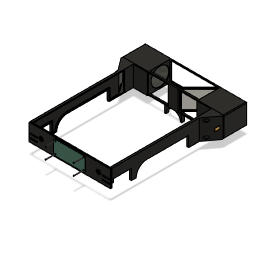
ARGlass (Autodesk Fusion 360 design; units mm, degrees)
Autodesk Fusion 360 part; units mm, degrees
note: some values were not read from the file. Chosen so that the rebuilt part matches the saved one: a direction; which face or edge a step refers to. Set by a fixed rule: which sketch regions a step uses; the direction of a hole.
(part 1 of 2)
sketch "スケッチ1" plane through (0, 0, 0) normal (0, 1, 0) x (1, 0, 0) in component "Display"
  line L0 (0, 0) -> (26.85, 0)
  line L1 (26.85, 0) -> (26.85, -29.55)
  line L2 (26.85, -29.55) -> (0, -29.55)
  line L3 (0, -29.55) -> (0, 0)
  dimension "d1" = 26.85
  dimension "d2" = 29.55
  constraint horizontal L0
  constraint vertical L1
  constraint horizontal L2
  constraint vertical L3
  constraint coincident L0.start L3.end
  measures "d1" distance of L0.start L0.end
  measures "d2" distance of L0.start L2.end
extrude "押し出し1" add sketch "スケッチ1" along normal blind 1.37 makes body 1 in component "Display"
sketch "スケッチ2" plane through (0, 1.37, 0) normal (0, 1, 0) x (-1, 0, 0) in component "Display"
  line L0 (0, 29.55) -> (-26.85, 29.55)
  line L1 (-26.85, 29.55) -> (-26.85, 0)
  line L2 (-26.85, 0) -> (0, 0)
  line L3 (0, 0) -> (0, 29.55)
  line L4 (-0.52, 0.55) -> (-26.32, 0.55)
  line L5 (-26.32, 0.55) -> (-26.32, 28.95)
  line L6 (-26.32, 28.95) -> (-0.52, 28.95)
  line L7 (-0.52, 28.95) -> (-0.52, 0.55)
  dimension "d5" = 25.8
  dimension "d6" = 28.4
  dimension "d7" = 0.55
  dimension "d8" = 0.53
  constraint horizontal L4
  constraint vertical L5
  constraint horizontal L6
  constraint vertical L7
  measures "d5" distance of L4.start L4.end
  measures "d6" distance of L4.start L6.end
  measures "d7" distance of L2 L4
  measures "d8" distance of L1 L5
extrude "押し出し2" add sketch "スケッチ2" along normal blind 0.36 separate body contours L4 L5 L6 L7 makes body 2 in component "Display"
sketch "スケッチ3" plane through (0, 1.37, 0) normal (0, 1, 0) x (-1, 0, 0) in component "Display"
  line L0 (0, 29.55) -> (-26.85, 29.55)
  line L1 (-26.85, 29.55) -> (-26.85, 0)
  line L2 (-26.85, 0) -> (0, 0)
  line L3 (0, 0) -> (0, 29.55)
  line L4 (-5.05, 28.95) -> (-23.05, 28.95)
  line L5 (-23.05, 28.95) -> (-23.05, 33.95)
  line L6 (-5.05, 33.95) -> (-5.05, 28.95)
  line L7 (-5.05, 33.95) -> (-10.8, 33.95)
  line L8 (-10.8, 33.95) -> (-10.8, 49.55)
  line L9 (-10.8, 49.55) -> (-17.3, 49.55)
  line L10 (-17.3, 49.55) -> (-17.3, 33.95)
  line L11 (-17.3, 33.95) -> (-23.05, 33.95)
  line L12 (-14.05, 28.95) -> (-14.05, 49.55) construction
  line L13 (-0.52, 28.95) -> (-26.32, 28.95)
  dimension "d11" = 6.5
  dimension "d12" = 10.8
  dimension "d13" = 18
  dimension "d14" = 20
  dimension "d15" = 5
  constraint horizontal L4
  constraint vertical L5
  constraint vertical L6
  constraint perpendicular L6 L7
  constraint perpendicular L7 L8
  constraint perpendicular L6 L9
  constraint perpendicular L9 L10
  constraint perpendicular L5 L11
  constraint midpoint L4 L12.start
  constraint midpoint L9 L12.end
  constraint vertical L12
  constraint collinear L4 L13
  constraint collinear L7 L11
  measures "d11" distance of L8.end L9.end
  measures "d12" distance of L3 L8
  measures "d13" distance of L5 L6
  measures "d14" distance of L0 L9
  measures "d15" distance of L4.end L5.end
extrude "押し出し3" add sketch "スケッチ3" against normal blind 0.3 separate body contours L0 L5 L6 L7 L8 L9 L10 L11 makes body 3 in component "Display"
sketch "スケッチ1 (2)" plane through (0, 0, 0) normal (0, 0, 1) x (1, 0, 0) in component "Lens"
  arc A0 (18.375, 0.3703) -> (0, 1.5) centre (0, -148.5) ccw
  line L0 (0, 0) -> (25.0146, 0) construction
  arc A1 (0, -1.5) -> (18.375, -0.3703) centre (0, 148.5) ccw
  line L1 (18.375, -0.3703) -> (18.375, 0.3703)
  line L2 (0, -1.5) -> (0, 1.5)
  line L3 (0, 1.5) -> (-2.5, 1.5) construction
  dimension "d18" = 150
  dimension "d19" = 3
  dimension "d20" = 18.375
  constraint coincident L0.start origin
  constraint horizontal L0
  constraint symmetric A0.start L0 A1.end
  constraint symmetric A0.end L0 A1.start
  constraint symmetric A0 L0 A1
  constraint coincident L0.start L2
  constraint perpendicular L2 L3
  constraint tangent A0 L3
  measures "d18" radius of A0
  measures "d19" distance of A0.end A1.start
  measures "d20" distance of L0.start L1
revolve "回転1" add sketch "スケッチ1 (2)" angle 360 about axis through (0, 1.75, 0) along (0, 1, 0) separate body makes body 4 in component "Lens"
sketch "スケッチ1 (3)" plane through (0, 0, 0) normal (0, 1, 0) x (1, 0, 0) in component "HalfMirror"
  line L0 (0, 0) -> (38, 0)
  line L1 (38, 0) -> (38, -54)
  line L2 (38, -54) -> (0, -54)
  line L3 (0, -54) -> (0, 0)
  dimension "d80" = 38
  dimension "d81" = 54
  constraint horizontal L0
  constraint vertical L1
  constraint horizontal L2
  constraint vertical L3
  constraint coincident L0.start L3.end
  measures "d80" distance of L0.start L0.end
  measures "d81" distance of L0.start L2.end
extrude "押し出し1'" add sketch "スケッチ1 (3)" along normal blind 0.5 separate body makes body 5 in component "HalfMirror"
sketch "スケッチ1 (4)" plane through (0, 0, 0) normal (0, 1, 0) x (1, 0, 0) in component "Pi Zero W"
  line L0 (3, 0) -> (62, 0)
  line L1 (65, -3) -> (65, -27)
  line L2 (62, -30) -> (3, -30)
  line L3 (0, -27) -> (0, -3)
  arc A0 (3, 0) -> (0, -3) centre (3, -3) ccw
  arc A1 (65, -3) -> (62, 0) centre (62, -3) ccw
  arc A2 (62, -30) -> (65, -27) centre (62, -27) ccw
  arc A3 (0, -27) -> (3, -30) centre (3, -27) ccw
  point P0 (65, 0)
  point P1 (0, -30)
  point P2 (3.5, -3.5)
  point P3 (61.5, -3.5)
  point P4 (3.5, -26.5)
  point P5 (61.5, -26.5)
  dimension "d140" = 65
  dimension "d141" = 30
  dimension "d142" = 3
  dimension "d143" = 3.5
  dimension "d144" = 3.5
  dimension "d147" = 58
  dimension "d148" = -23
  constraint horizontal L0
  constraint vertical L1
  constraint horizontal L2
  constraint vertical L3
  constraint coincident origin L0
  constraint coincident origin L3
  constraint tangent L0 A0
  constraint tangent L3 A0
  constraint coincident P0 L0
  constraint coincident P0 L1
  constraint tangent L0 A1
  constraint tangent L1 A1
  constraint equal A0 A1
  constraint tangent L1 A2
  constraint tangent L2 A2
  constraint equal A0 A2
  constraint coincident P1 L2
  constraint coincident P1 L3
  constraint tangent L2 A3
  constraint tangent L3 A3
  constraint equal A0 A3
  measures "d140" distance of origin P0
  measures "d141" distance of origin P1
  measures "d142" radius of A0
  measures "d143" distance of L0 P2
  measures "d144" distance of L3 P2
extrude "押し出し1''" add sketch "スケッチ1 (4)" along normal blind 1 separate body makes body 6 in component "Pi Zero W"
hole "穴1" at (3.5, 0, 26.5) at (3.5, 0, 3.5) at (61.5, 0, 3.5) at (61.5, 0, 26.5) direction (0, 1, 0) diameter 2.5 end through all bodies 6 in component "Pi Zero W"
sketch "スケッチ1 (5)" plane through (0, 0, 0) normal (0, 1, 0) x (1, 0, 0) in component "FrontUnit"
  line L0 (0, 3) -> (7.1716, 3)
  line L1 (0, 0) -> (0, 3)
  line L2 (49.1716, 45) -> (52.1716, 48)
  line L3 (103, 0) -> (0, 0)
  line L4 (53, 46) -> (53, 3)
  line L5 (10, 3) -> (53, 3)
  line L6 (103, 0) -> (103, 48)
  line L7 (52.1716, 48) -> (103, 48)
  line L8 (10, 3) -> (53, 46)
  line L9 (31.5, 24.5) -> (31.5, 0) construction
  line L10 (53, 46) -> (50.1716, 46) construction
  line L11 (52.1716, 48) -> (0, 48)
  line L12 (0, 48) -> (0, 45)
  line L13 (0, 45) -> (49.1716, 45)
  line L14 (7.1716, 3) -> (49.1716, 45)
  dimension "d23" = 3
  dimension "d24" = 31.5
  dimension "d27" = 43
  dimension "d28" = 2
  dimension "d29" = 50
  dimension "d55" = 3
  dimension "d56" = 45
  dimension "d57" = 2
  constraint horizontal L0
  constraint horizontal L3
  constraint vertical L1
  constraint perpendicular L4 L5
  constraint perpendicular L6 L7
  constraint horizontal L7
  constraint horizontal L5
  constraint coincident L1.start L3.end
  constraint collinear L0 L5
  constraint midpoint L8 L9.start
  constraint coincident L3 L9.end
  constraint perpendicular L3 L9
  constraint coincident L2 L10.end
  constraint horizontal L10
  constraint coincident L4.start L10
  constraint perpendicular L4 L11
  constraint perpendicular L11 L12
  constraint perpendicular L12 L13
  constraint collinear L1 L12
  constraint parallel L8 L14
  constraint parallel L2 L8
  constraint coincident L4.start L8.end
  measures "d23" distance of L0.start L1.start
  measures "d24" distance of L1 L9
  measures "d27" distance of L4.start L4.end
  measures "d28" distance of L4.start L7
  measures "d29" distance of L4 L6
  measures "d55" distance of L11.end L12.end
  measures "d56" angle of L5 L8
  measures "d57" distance of L8 L14
extrude "押し出し1'''" add sketch "スケッチ1 (5)" along normal blind 2 separate body makes body 7 in component "FrontUnit"
sketch "スケッチ2 (2)" plane through (53, 0, 0) normal (-1, 0, 0) x (0, 0, 1) in component "FrontUnit"
  line L0 (-46, 0) -> (-3, 0)
  line L1 (-3, 0) -> (-3, 2)
  line L2 (-3, 2) -> (-46, 2)
  line L3 (-46, 2) -> (-3, 2)
  line L4 (-24.5, 2) -> (-24.5, 21) construction
  line L5 (-48, 40) -> (-48, 2)
  line L6 (-48, 2) -> (-46, 2)
  line L7 (0, 40) -> (0, 2)
  line L8 (-3, 2) -> (0, 2)
  circle A0 centre (-24.5, 21) radius 19
  line L9 (-48, 40) -> (0, 40)
  line L10 (-46, 2) -> (-46, 0)
  point P0 (0, 2)
  point P1 (-48, 2)
  dimension "d36" = 38
  constraint midpoint L3 L4.start
  constraint vertical L4
  constraint coincident L2.end L3.start
  constraint perpendicular L3 L7
  constraint coincident L1.end L2.start
  constraint perpendicular L7 L8
  constraint coincident P0 L7.end
  constraint coincident L4.end A0.centre
  constraint tangent L2 A0
  constraint tangent A0 L9
  constraint horizontal L9
  constraint vertical L5
  constraint coincident L5 P1
  constraint coincident L6 P1
  measures "d36" diameter of A0
extrude "押し出し2'" add sketch "スケッチ2 (2)" along normal blind 2 contours L2 L3 L5 L6 A0 L9 | L2 L3 L7 L8 A0 L9 bodies 7 in component "FrontUnit"
sketch "スケッチ3 (2)" plane through (103, 0, 0) normal (1, 0, 0) x (0, 0, -1) in component "FrontUnit"
  line L0 (0, 0) -> (48, 0)
  line L1 (48, 0) -> (48, 2)
  line L2 (48, 2) -> (0, 2)
  line L3 (0, 2) -> (0, 0)
  line L4 (0, 0) -> (48, 0)
  line L5 (48, 0) -> (48, 40)
  line L6 (48, 40) -> (0, 40)
  line L7 (0, 40) -> (0, 0)
  point P0 (48, 40)
  constraint horizontal L4
  constraint vertical L5
  constraint horizontal L6
  constraint vertical L7
  constraint coincident L0.start L3.end
  constraint coincident P0 L5.end
extrude "押し出し3'" add sketch "スケッチ3 (2)" along normal blind 2 bodies 7 in component "FrontUnit"
sketch "スケッチ4" plane through (103, 0, 0) normal (-1, 0, 0) x (0, 0, 1) in component "FrontUnit"
  line L0 (-48, 2) -> (0, 2)
  line L1 (0, 2) -> (0, 40)
  line L2 (0, 40) -> (-48, 40)
  line L3 (-48, 40) -> (-48, 2)
  line L4 (-15.205, 34.675) -> (-45.255, 34.675)
  line L5 (-45.255, 34.675) -> (-45.255, 7.325)
  line L6 (-45.255, 7.325) -> (-15.205, 7.325)
  line L7 (-15.205, 7.325) -> (-15.205, 34.675) construction
  line L8 (-15.205, 34.675) -> (-45.255, 7.325) construction
  line L9 (-45.255, 34.675) -> (-15.205, 7.325) construction
  arc A0 (-24.5, 2) -> (-24.5, 40) centre (-24.5, 21) ccw construction
  arc A1 (-24.5, 40) -> (-24.5, 2) centre (-24.5, 21) ccw construction
  line L10 (-15.205, 34.675) -> (0, 34.675)
  line L11 (-15.205, 7.325) -> (0, 7.325)
  line L12 (-30.23, 21) -> (-24.5, 21) construction
  point P0 (-30.23, 21)
  dimension "d39" = 30.05
  dimension "d40" = 27.35
  dimension "d88" = 5.73
  constraint horizontal L4
  constraint perpendicular L4 L5
  constraint parallel L4 L6
  constraint parallel L5 L7
  constraint coincident L8 P0
  constraint coincident L9 P0
  constraint coincident L1 L10.end
  constraint perpendicular L1 L10
  constraint coincident L1 L11.end
  constraint perpendicular L1 L11
  constraint coincident P0 L12.start
  constraint coincident A0.centre A1.centre
  constraint horizontal L12
  measures "d39" distance of L5.end L6.end
  measures "d40" distance of L4.end L5.end
  measures "d88" distance of P0 A0.centre
extrude "押し出し4" add sketch "スケッチ4" along normal blind 1.3 contours L0 L1 L2 L3 L4 L5 L6 L10 L11 bodies 7 in component "FrontUnit"
sketch "スケッチ5" plane through (0, 0, -48) normal (0, 0, -1) x (-1, 0, 0) in component "FrontUnit"
  line L0 (-105, 0) -> (0, 0)
  line L1 (0, 2) -> (-51, 2)
  line L2 (-51, 2) -> (-51, 40)
  line L3 (-51, 40) -> (-53, 40)
  line L4 (-53, 40) -> (-53, 2)
  line L5 (-53, 2) -> (-101.7, 2)
  line L6 (-101.7, 2) -> (-101.7, 40)
  line L7 (-101.7, 40) -> (-105, 40)
  line L8 (-105, 40) -> (-105, 0)
  line L9 (-101.7, 40) -> (-101.7, 2)
  line L10 (-101.7, 2) -> (-53, 2)
  line L11 (-53, 40) -> (-53, 2)
  line L12 (-101.7, 40) -> (-53, 40)
  line L13 (0, 0) -> (0, 2)
  constraint coincident L6.end L7.start
  constraint coincident L3.end L4.start
extrude "押し出し5" add sketch "スケッチ5" against normal blind 2 contours L4 L5 L6 L9 L10 L11 L12 bodies 7 in component "FrontUnit"
sketch "スケッチ6" plane through (0, 40, 0) normal (0, 1, 0) x (-1, 0, 0) in component "FrontUnit"
  line L0 (-105, -48) -> (-51, -48)
  line L1 (-51, -48) -> (-51, -24.5)
  line L2 (-51, -24.5) -> (-53, -24.5)
  line L3 (-53, -24.5) -> (-53, -46)
  line L4 (-53, -46) -> (-101.7, -46)
  line L5 (-101.7, -46) -> (-101.7, 0)
  line L6 (-101.7, 0) -> (-105, 0)
  line L7 (-105, 0) -> (-105, -48)
  line L8 (-105, -48) -> (-51, -48)
  line L9 (-105, -48) -> (-105, 0)
  line L10 (-51, -24.5) -> (-51, -48)
  line L11 (-51, 0) -> (-51, -24.5)
  line L12 (-53, 0) -> (-51, 0)
  line L13 (-53, 0) -> (-101.7, 0)
  line L14 (-105, 0) -> (-101.7, 0)
extrude "押し出し6" add sketch "スケッチ6" along normal blind 2 bodies 7 in component "FrontUnit"
sketch "スケッチ7" plane through (0, 2, 0) normal (0, -1, 0) x (1, 0, 0) in component "FrontUnit"
  line L0 (53, -3) -> (51, -3)
  line L1 (51, -3) -> (51, -24.5)
  line L2 (53, -24.5) -> (53, -3)
  line L3 (51, -24.5) -> (51, -3)
  line L4 (53, -46) -> (53, -3)
  line L5 (51, -44) -> (51, -24.5)
  line L6 (53, -46) -> (51, -44)
  line L7 (51, -3) -> (53, -3)
  constraint coincident L4.start L6.start
  constraint coincident L5.start L6.end
  constraint coincident L0.end L1.start
  constraint coincident L0.start L2.end
extrude "押し出し7" add sketch "スケッチ7" along normal blind 2 bodies 7 in component "FrontUnit"
sketch "スケッチ8" plane through (0, 42, 0) normal (0, 1, 0) x (-1, 0, 0) in component "FrontUnit"
  line L0 (-105, -48) -> (-51, -48)
  line L1 (-51, -48) -> (-51, 0)
  line L2 (-51, 0) -> (-105, 0)
  line L3 (-105, 0) -> (-105, -48)
  line L4 (-51, -44) -> (-51, -48)
  line L5 (-51, -48) -> (0, -48)
  line L6 (-7.1716, -3) -> (0, -3)
  line L7 (0, -3) -> (0, 0)
  line L8 (0, 0) -> (-51, 0)
  line L9 (-51, 0) -> (-51, -3)
  line L10 (-51, -3) -> (-10, -3)
  line L11 (0, -48) -> (0, -45)
  line L12 (0, -45) -> (-49.1716, -45)
  line L13 (-49.1716, -45) -> (-7.1716, -3)
  line L14 (-10, -3) -> (-51, -44)
extrude "押し出し8" add sketch "スケッチ8" against normal blind 2 contours L1 L4 L5 L6 L7 L8 L9 L10 L11 L12 L13 L14 bodies 7 in component "FrontUnit"
sketch "スケッチ9" plane through (0, 2, 0) normal (0, 1, 0) x (-1, 0, 0) in component "FrontUnit"
  line L0 (-51, -44) -> (-51, -48)
  line L1 (-51, -48) -> (0, -48)
  line L2 (-7.1716, -3) -> (0, -3)
  line L3 (0, -3) -> (0, 0)
  line L4 (0, 0) -> (-51, 0)
  line L5 (-51, 0) -> (-51, -3)
  line L6 (-51, -3) -> (-10, -3)
  line L7 (0, 0) -> (-10, 0)
  line L8 (-10, 0) -> (-10, -3)
  line L9 (-10, -3) -> (0, -3)
  line L10 (0, -3) -> (0, 0)
  line L11 (0, -48) -> (0, -45)
  line L12 (0, -45) -> (-49.1716, -45)
  line L13 (-49.1716, -45) -> (-7.1716, -3)
  line L14 (-10, -3) -> (-51, -44)
  dimension "d51" = 10
  dimension "d52" = 3
  constraint horizontal L7
  constraint vertical L8
  constraint horizontal L9
  constraint vertical L10
  constraint coincident L3.end L4.start
  measures "d51" distance of L6.end L2.end
  measures "d52" distance of L3.end L2.end
extrude "押し出し9" add sketch "スケッチ9" along normal up to near side of body 7 contours L2 L3 L4 L7 L8 L9 L10 bodies 7 in component "FrontUnit"
sketch "スケッチ10" plane through (3.5, 0, 3.5) normal (0.707107, 0, 0.707107) x (0.707107, 0, -0.707107) in component "FrontUnit"
  line L0 (67.1751, 42) -> (9.1924, 42)
  line L1 (9.1924, 42) -> (9.1924, 40)
  line L2 (9.1924, 40) -> (67.1751, 40)
  line L3 (67.1751, 40) -> (67.1751, 42)
  line L4 (12.1924, 39) -> (64.1751, 39)
  line L5 (64.1751, 39) -> (64.1751, 3)
  line L6 (64.1751, 3) -> (12.1924, 3)
  line L7 (12.1924, 3) -> (12.1924, 39)
  line L8 (9.1924, 42) -> (67.1751, 42)
  line L9 (9.1924, 0) -> (67.1751, 0)
  line L10 (6.1924, 42) -> (6.1924, 0)
  line L11 (6.1924, 0) -> (9.1924, 0)
  line L12 (6.1924, 42) -> (9.1924, 42)
  line L13 (67.1751, 42) -> (70.1751, 42)
  line L14 (70.1751, 42) -> (70.1751, 0)
  line L15 (70.1751, 0) -> (67.1751, 0)
  dimension "d62" = 3
  dimension "d63" = 3
  dimension "d64" = 3
  dimension "d65" = 3
  dimension "d68" = 3
  dimension "d69" = 3
  constraint horizontal L4
  constraint vertical L5
  constraint horizontal L6
  constraint vertical L7
  constraint vertical L10
  constraint coincident L9.start L11.end
  constraint perpendicular L10 L11
  constraint coincident L0.end L1.start
  constraint horizontal L12
  constraint coincident L0.start L3.end
  constraint perpendicular L3 L13
  constraint perpendicular L8 L14
  constraint coincident L9.end L15.end
  constraint perpendicular L14 L15
  measures "d62" distance of L0 L4
  measures "d63" distance of L6 L9
  measures "d64" distance of L10.start L0.end
  measures "d65" distance of L0.start L13.end
  measures "d68" distance of L7 L0.end
  measures "d69" distance of L5 L0.start
extrude "押し出し10" add sketch "スケッチ10" against normal blind 2 bodies 7 in component "FrontUnit"
sketch "スケッチ12" plane through (3.5, 0, 3.5) normal (0.707107, 0, 0.707107) x (0.707107, 0, -0.707107) in component "FrontUnit"
  line L0 (64.1751, 3) -> (12.1924, 3)
  line L1 (12.1924, 3) -> (12.1924, 39)
  line L2 (12.1924, 39) -> (64.1751, 39)
  line L3 (64.1751, 39) -> (64.1751, 3)
  line L4 (67.1751, 0) -> (67.1751, 42)
  line L5 (67.1751, 42) -> (9.1924, 42)
  line L6 (9.1924, 42) -> (9.1924, 40)
  line L7 (9.1924, 40) -> (9.1924, 2)
  line L8 (9.1924, 2) -> (9.1924, 0)
  line L9 (9.1924, 0) -> (67.1751, 0)
  line L10 (10.6924, 40.5) -> (65.6751, 40.5)
  line L11 (65.6751, 40.5) -> (65.6751, 1.5)
  line L12 (65.6751, 1.5) -> (10.6924, 1.5)
  line L13 (10.6924, 1.5) -> (10.6924, 40.5)
  line L14 (12.1924, 39) -> (12.1924, 3)
  line L15 (12.1924, 39) -> (64.1751, 39)
  line L16 (64.1751, 3) -> (64.1751, 39)
  line L17 (64.1751, 3) -> (12.1924, 3)
  line L18 (64.1751, 3) -> (64.1751, 39)
  line L19 (64.1751, 39) -> (64.1751, 3)
  dimension "d235" = 1.5
  dimension "d236" = 1.5
  dimension "d237" = 1.5
  dimension "d238" = 1.5
  constraint horizontal L10
  constraint vertical L11
  constraint horizontal L12
  constraint vertical L13
  measures "d235" distance of L10 L15
  measures "d236" distance of L13 L14
  measures "d237" distance of L11 L19
  measures "d238" distance of L0 L12
extrude "押し出し13" cut sketch "スケッチ12" against normal blind 0.5 contours L10 L11 L12 L13 bodies 7 in component "FrontUnit"
sketch "スケッチ11" plane through (0, 0, 0) normal (0, 0, 1) x (1, 0, 0) in component "FrontUnit"
  line L0 (10, 40) -> (51, 40)
  line L1 (51, 40) -> (51, 2)
  line L2 (51, 2) -> (10, 2)
  line L3 (10, 2) -> (10, 40)
  line L4 (0, 42) -> (0, 0)
  line L5 (0, 0) -> (105, 0)
  line L6 (105, 0) -> (105, 42)
  line L7 (105, 42) -> (0, 42)
  line L8 (53, 40) -> (101.7, 40)
  line L9 (101.7, 40) -> (101.7, 34.675)
  line L10 (101.7, 34.675) -> (103, 34.675)
  line L11 (103, 34.675) -> (103, 7.325)
  line L12 (103, 7.325) -> (101.7, 7.325)
  line L13 (101.7, 7.325) -> (101.7, 2)
  line L14 (101.7, 2) -> (53, 2)
  line L15 (53, 2) -> (53, 40)
  line L16 (85.3, 40) -> (94.7, 40)
  line L17 (94.7, 40) -> (94.7, 36.15)
  line L18 (85.3, 36.15) -> (85.3, 40)
  arc A0 (85.3, 36.15) -> (94.7, 36.15) centre (90, 36.15) ccw
  line L19 (91.6454, 33.3) -> (93.2909, 36.15)
  line L20 (93.2909, 36.15) -> (91.6454, 39)
  line L21 (91.6454, 39) -> (88.3546, 39)
  line L22 (88.3546, 39) -> (86.7091, 36.15)
  line L23 (86.7091, 36.15) -> (88.3546, 33.3)
  line L24 (88.3546, 33.3) -> (91.6454, 33.3)
  line L25 (0, 21) -> (105, 21) construction
  line L26 (85.3, 5.85) -> (85.3, 2)
  arc A1 (94.7, 5.85) -> (85.3, 5.85) centre (90, 5.85) ccw
  line L27 (94.7, 2) -> (94.7, 5.85)
  line L28 (85.3, 2) -> (94.7, 2)
  line L29 (93.2909, 5.85) -> (91.6454, 3)
  line L30 (91.6454, 8.7) -> (93.2909, 5.85)
  line L31 (88.3546, 8.7) -> (91.6454, 8.7)
  line L32 (86.7091, 5.85) -> (88.3546, 8.7)
  line L33 (88.3546, 3) -> (86.7091, 5.85)
  line L34 (91.6454, 3) -> (88.3546, 3)
  point P0 (90, 36.15)
  dimension "d89" = 5.7
  dimension "d90" = 1
  dimension "d91" = 90
  dimension "d92" = 9.4
  constraint horizontal L16
  constraint vertical L17
  constraint vertical L18
  constraint coincident L8 L16.start
  constraint tangent L18 A0
  constraint tangent L17 A0
  constraint coincident P0 A0.centre
  constraint midpoint L4 L25.start
  constraint midpoint L6 L25.end
  constraint symmetric L16.start L25 L26.end
  constraint symmetric L16.end L25 L27.start
  constraint symmetric L17.end L25 A1.start
  constraint symmetric L18.start L25 L26.start
  constraint symmetric A0 L25 A1
  constraint symmetric L19.start L25 L30.start
  constraint symmetric L19.end L25 L29.start
  constraint symmetric L20.end L25 L29.end
  constraint symmetric L21.end L25 L33.start
  constraint symmetric L22.end L25 L32.start
  constraint symmetric L23.end L25 L31.start
  measures "d89" distance of L21 L24
  measures "d90" distance of L16 L21
  measures "d91" distance of L4 P0
  measures "d92" distance of L16.start L16.end
extrude "押し出し11" add sketch "スケッチ11" against normal blind 4.5 contours L8 L16 L17 L18 A0 | L14 L26 A1 L27 L28 | L19 L20 L21 L22 L23 L24 | L29 L30 L31 L32 L33 L34 bodies 7 in component "FrontUnit"
extrude "押し出し12" cut sketch "スケッチ11" against normal blind 3 contours L19 L20 L21 L22 L23 L24 | L29 L30 L31 L32 L33 L34 bodies 7 in component "FrontUnit"
ref_plane "作業平面1" through (80, 0, 0) normal (1, 0, 0) x (0, 1, 0) in component "SideUnit"
sketch "スケッチ1 (6)" plane through (80, 0, 0) normal (1, 0, 0) x (0, 0, -1) in component "SideUnit"
  line L0 (0, 0) -> (-30, 0)
  line L1 (-30, 42) -> (0, 42)
  line L2 (0, 42) -> (0, 0)
  line L3 (0, 42) -> (48, 42) construction
  line L4 (-30, 0) -> (-30, 42)
  dimension "d98" = 30
  constraint horizontal L0
  constraint horizontal L1
  constraint vertical L2
  constraint coincident L0.start L2.end
  constraint coincident L1.end L2.start
  constraint vertical L4
  measures "d98" distance of L0.start L0.end
extrude "押し出し1''''" add sketch "スケッチ1 (6)" along normal blind 2 separate body makes body 8 in component "SideUnit"
sketch "スケッチ2 (3)" plane through (0, 0, 0) normal (0, 0, 1) x (1, 0, 0) in component "SideUnit"
  line L0 (93.2909, 36.15) -> (91.6454, 33.3)
  line L1 (91.6454, 33.3) -> (88.3546, 33.3)
  line L2 (88.3546, 33.3) -> (86.7091, 36.15)
  line L3 (86.7091, 36.15) -> (88.3546, 39)
  line L4 (88.3546, 39) -> (91.6454, 39)
  line L5 (91.6454, 39) -> (93.2909, 36.15)
  line L6 (91.6454, 8.7) -> (93.2909, 5.85)
  line L7 (93.2909, 5.85) -> (91.6454, 3)
  line L8 (91.6454, 3) -> (88.3546, 3)
  line L9 (88.3546, 3) -> (86.7091, 5.85)
  line L10 (86.7091, 5.85) -> (88.3546, 8.7)
  line L11 (88.3546, 8.7) -> (91.6454, 8.7)
  line L12 (10, 40) -> (51, 40)
  line L13 (51, 40) -> (51, 2)
  line L14 (51, 2) -> (10, 2)
  line L15 (10, 2) -> (10, 40)
  line L16 (0, 42) -> (0, 0)
  line L17 (0, 0) -> (105, 0)
  line L18 (105, 0) -> (105, 42)
  line L19 (105, 42) -> (0, 42)
  line L20 (94.7, 40) -> (101.7, 40)
  line L21 (101.7, 40) -> (101.7, 34.675)
  line L22 (101.7, 7.325) -> (101.7, 2)
  line L23 (101.7, 2) -> (94.7, 2)
  line L24 (94.7, 2) -> (94.7, 5.85)
  arc A0 (94.7, 5.85) -> (85.3, 5.85) centre (90, 5.85) ccw
  line L25 (85.3, 5.85) -> (85.3, 2)
  line L26 (85.3, 2) -> (53, 2)
  line L27 (53, 2) -> (53, 40)
  line L28 (53, 40) -> (85.3, 40)
  line L29 (85.3, 40) -> (85.3, 36.15)
  arc A1 (85.3, 36.15) -> (94.7, 36.15) centre (90, 36.15) ccw
  line L30 (94.7, 36.15) -> (94.7, 40)
  line L31 (51, 42) -> (105, 42)
  line L32 (105, 0) -> (51, 0)
  line L33 (51, 0) -> (51, 42)
  line L34 (53, 40) -> (53, 2) construction
  line L35 (105, 0) -> (105, 42)
  line L36 (101.7, 34.675) -> (101.7, 40)
  line L37 (101.7, 2) -> (101.7, 7.325)
  line L38 (53, 40) -> (82, 40)
  line L39 (82, 42) -> (82, 0) construction
  line L40 (53, 2) -> (82, 2)
  line L41 (82, 40) -> (101.7, 40)
  line L42 (82, 2) -> (101.7, 2)
  line L43 (82, 2) -> (82, 40)
  line L44 (101.7, 34.675) -> (101.7, 7.325)
  dimension "d105" = 2
  constraint horizontal L31
  constraint horizontal L32
  constraint vertical L33
  constraint coincident L19 L31.start
  constraint coincident L18.end L19.start
  constraint coincident L17.end L18.start
  constraint coincident L27.end L28.start
  constraint coincident L28 L38.end
  constraint coincident L38.end L39
  constraint coincident L26.end L27.start
  constraint coincident L39 L40.end
  constraint coincident L26 L40.end
  constraint coincident L20.end L21.start
  constraint coincident L22.end L23.start
  constraint coincident L21.end L36.start
  constraint coincident L22.start L37.end
  measures "d105" distance of L33 L34
extrude "押し出し2''" add sketch "スケッチ2 (3)" along normal blind 2 contours L13 L17 L18 L19 L31 L32 L33 L35 | L26 L27 L28 L38 L40 L43 bodies 8 in component "SideUnit"
sketch "スケッチ3 (3)" plane through (0, 0, 0) normal (0, -1, 0) x (1, 0, 0) in component "SideUnit"
  line L0 (82, 2) -> (82, 30)
  line L1 (82, 30) -> (80, 30)
  line L2 (80, 30) -> (80, 2)
  line L3 (80, 2) -> (51, 2)
  line L4 (51, 2) -> (51, 0)
  line L5 (82, 30) -> (82, 2)
  line L6 (105, 2) -> (84, 30)
  line L7 (84, 30) -> (82, 30)
  line L8 (105, 2) -> (82, 2)
  dimension "d108" = 2
  constraint coincident L0.end L1.start
  constraint horizontal L7
  constraint coincident L6.start L8.start
  measures "d108" distance of L6.end L0.end
extrude "押し出し3''" add sketch "スケッチ3 (3)" against normal blind 2 bodies 8 in component "SideUnit"
sketch "スケッチ7 (2)" plane through (0, 42, 0) normal (0, 1, 0) x (-1, 0, 0) in component "SideUnit"
  line L0 (-80, 2) -> (-80, 30)
  line L1 (-80, 30) -> (-82, 30)
  line L2 (-82, 30) -> (-82, 2)
  line L3 (-82, 2) -> (-105, 2)
  line L4 (-105, 2) -> (-105, 0)
  line L5 (-105, 0) -> (-51, 0)
  line L6 (-51, 0) -> (-51, 2)
  line L7 (-51, 2) -> (-80, 2)
  line L8 (-105, 2) -> (-101.7, 2)
  line L9 (-82, 0) -> (-82, 30)
  line L10 (-82, 30) -> (-84, 30)
  line L11 (-84, 30) -> (-105, 2)
  line L12 (-101.7, 0) -> (-82, 0)
  line L13 (-101.7, 2) -> (-101.7, 0)
extrude "押し出し7'" add sketch "スケッチ7 (2)" against normal blind 2 contours L2 L3 L8 L9 L10 L11 bodies 8 in component "SideUnit"
ref_plane "作業平面2" through (82, 0, 0) normal (1, 0, 0) x (0, 1, 0) in component "SideUnit"
sketch "スケッチ10 (2)" plane through (82, 0, 0) normal (1, 0, 0) x (0, 0, -1) in component "SideUnit"
  line L0 (-30, 40) -> (-30, 2)
  line L1 (-30, 42) -> (-30, 40)
  line L2 (-30, 0) -> (-30, 2)
  line L3 (-30, 42) -> (-50, 42)
  line L4 (-50, 42) -> (-50, 0)
  line L5 (-50, 0) -> (-30, 0)
  line L6 (-30, 40) -> (-50, 40)
  line L7 (-30, 2) -> (-50, 2)
  line L8 (-50, 42) -> (-170, 42)
  line L9 (-170, 42) -> (-170, 22)
  line L10 (-138, 24) -> (-50, 24)
  line L11 (-50, 40) -> (-170, 40)
  line L12 (-52, 22) -> (-52, 0)
  line L13 (-52, 0) -> (-50, 0)
  arc A0 (-138, 22) -> (-160, 0) centre (-138, 0) ccw
  line L14 (-160, 22) -> (-160, 0) construction
  line L15 (-160, 0) -> (-52, 0) construction
  line L16 (-160, 0) -> (-170, 0)
  line L17 (-170, 0) -> (-170, 22)
  arc A1 (-138, 24) -> (-161.9165, 2) centre (-138, 0) ccw
  line L18 (-161.9165, 2) -> (-168, 2)
  line L19 (-168, 2) -> (-168, 22)
  line L20 (-170, 22) -> (-168, 22) construction
  line L21 (-138, 22) -> (-50, 22)
  line L22 (-170, 42) -> (-210, 42)
  line L23 (-210, 42) -> (-210, 22)
  line L24 (-210, 22) -> (-170, 22)
  line L25 (-170, 40) -> (-210, 40)
  line L26 (-210, 24) -> (-168, 24)
  line L27 (-168, 22) -> (-168, 24)
  dimension "d126" = 20
  dimension "d132" = 20
  dimension "d133" = 120
  dimension "d134" = 2
  dimension "d137" = 160
  dimension "d138" = 2
  dimension "d139" = 2
  dimension "d168" = 40
  dimension "d169" = 2
  constraint coincident L1.start L3.start
  constraint perpendicular L1 L3
  constraint perpendicular L3 L4
  constraint coincident L2.start L5.end
  constraint perpendicular L2 L5
  constraint coincident L0.start L1.end
  constraint coincident L4 L6.end
  constraint perpendicular L4 L6
  constraint coincident L0.end L2.end
  constraint coincident L4 L7.end
  constraint perpendicular L4 L7
  constraint perpendicular L4 L8
  constraint perpendicular L3 L9
  constraint coincident L4 L21.end
  constraint perpendicular L4 L20
  constraint coincident L4 L10.end
  constraint perpendicular L4 L10
  constraint coincident L9 L11.end
  constraint perpendicular L9 L11
  constraint coincident L12.start L20
  constraint perpendicular L12 L20
  constraint perpendicular L4 L13
  constraint tangent A0 L20
  constraint coincident A0.start L20
  constraint coincident L14.start L20
  constraint vertical L14
  constraint tangent A0 L14
  constraint horizontal L15
  constraint perpendicular L14 L16
  constraint perpendicular L17 L20
  constraint collinear L20 L21
  constraint perpendicular L9 L22
  constraint perpendicular L22 L23
  constraint horizontal L24
  constraint coincident L23 L25.end
  constraint perpendicular L23 L25
  constraint coincident L23 L26.start
  constraint perpendicular L9 L26
  constraint collinear L19 L27
  measures "d126" distance of L1.start L3.end
  measures "d132" distance of L8 L20
  measures "d133" distance of L3.end L8.end
  measures "d134" distance of L4 L12
  measures "d137" distance of origin L14
  measures "d139" distance of L10 L21
  measures "d168" distance of L8.end L22.end
  measures "d169" distance of L24 L26
extrude "押し出し10'" add sketch "スケッチ10 (2)" along normal blind 2 bodies 8 in component "SideUnit"
extrude "押し出し11'" add sketch "スケッチ10 (2)" against normal up to surface (2 mm away) contours L1 L3 L4 L6 | L2 L4 L5 L7 | L4 L8 L9 L11 | L4 L12 L13 L21 | L4 L9 L10 A0 L16 L17 A1 L18 L19 L21 L26 L27 | L9 L22 L23 L25 | L9 L23 L24 L26 bodies 8 in component "SideUnit"
sketch "スケッチ12 (2)" plane through (0, 0, 0) normal (0, 0, -1) x (-1, 0, 0) in component "SideUnit"
  line L0 (-82, 40) -> (-82, 2)
  line L1 (-82, 2) -> (-101.7, 2)
  line L2 (-101.7, 2) -> (-101.7, 40)
  line L3 (-101.7, 40) -> (-82, 40)
  line L4 (-51, 42) -> (-105, 42)
  line L5 (-105, 42) -> (-105, 0)
  line L6 (-105, 0) -> (-51, 0)
  line L7 (-51, 0) -> (-51, 42)
  arc A0 (-94.7, 36.15) -> (-85.3, 36.15) centre (-90, 36.15) ccw
  line L8 (-94.7, 40) -> (-94.7, 36.15)
  line L9 (-85.3, 36.15) -> (-85.3, 40)
  line L10 (-94.7, 2) -> (-94.7, 5.85)
  arc A1 (-85.3, 5.85) -> (-94.7, 5.85) centre (-90, 5.85) ccw
  line L11 (-85.3, 5.85) -> (-85.3, 2)
  line L12 (-85.3, 40) -> (-94.7, 40)
  line L13 (-85.3, 2) -> (-94.7, 2)
  circle A2 centre (-90, 36.15) radius 1.6
  circle A3 centre (-90, 5.85) radius 1.6
  dimension "d156" = 3.2
  constraint coincident L9.end L12.start
  constraint coincident L8.start L12.end
  constraint coincident L11.end L13.start
  constraint coincident L10.start L13.end
  constraint concentric A0 A2
  constraint concentric A1 A3
  constraint equal A2 A3
  measures "d156" diameter of A2
extrude "押し出し13'" add sketch "スケッチ12 (2)" against normal blind 3 contours L3 A0 L8 L9 L12 | L1 L10 A1 L11 L13 bodies 8 in component "SideUnit"
sketch "スケッチ11 (2)" plane through (0, 2, 0) normal (0, 1, 0) x (-1, 0, 0) in component "SideUnit"
  line L0 (-85.3, 0) -> (-82, 0)
  line L1 (-82, 0) -> (-82, 30)
  line L2 (-82, 30) -> (-84, 30)
  line L3 (-84, 30) -> (-105, 2)
  line L4 (-105, 2) -> (-101.7, 2)
  line L5 (-101.7, 2) -> (-101.7, 0)
  line L6 (-84, 30) -> (-105, 2)
  line L7 (-101.7, 2) -> (-105, 2)
  line L8 (-82, 30) -> (-84, 30)
  line L9 (-82, 30) -> (-101.7, 2)
  line L10 (-85.3, 3) -> (-85.3, 0)
  line L11 (-94.7, 0) -> (-94.7, 3)
  line L12 (-94.7, 3) -> (-85.3, 3)
  line L13 (-101.7, 0) -> (-94.7, 0)
  constraint coincident L1.end L2.start
  constraint coincident L4.end L5.start
extrude "押し出し12'" add sketch "スケッチ11 (2)" along normal up to surface (38 mm away) contours L2 L3 L4 L6 L7 L8 L9 bodies 8 in component "SideUnit"
ref_plane "作業平面3" through (0, 0, 6) normal (0, 0, 1) x (1, 0, 0) in component "SideUnit"
sketch "スケッチ13" plane through (0, 0, 6) normal (0, 0, 1) x (1, 0, 0) in component "SideUnit"
  point P0 (90, 36.15)
  point P1 (90, 5.85)
hole "穴1'" at (90, 36.15, 6) at (90, 5.85, 6) direction (0, 0, 1) diameter 6 depth 30 tip angle 180 bodies 8 in component "SideUnit"
fillet "フィレット1" radius 1.5 5 edges at (105, 42, -24) (105, 0, -24) (105, 21, -48) (52.5, 42, -48) (52.5, 0, -48) on bodies 7 in component "FrontUnit"
mirror "ミラー1" about plane through (0, 0, 0) normal (1, 0, 0) of bodies 7 merged in component "FrontUnit"
mirror "コンポーネントをミラー化1" about plane through (0, 0, 0) normal (0, 0, 1) of bodies 4 makes body 9 in component "Lens(ミラー)"
mirror "コンポーネントをミラー化1'" about plane through (0, 0, 0) normal (0, 0, 1) of bodies 5 makes body 10 in component "HalfMirror(ミラー)"
mirror "コンポーネントをミラー化1''" about plane through (0, 0, 0) normal (0, 0, 1) of bodies 1 2 3 makes body 11 at (8.95, 0, -9.85) makes body 12 at (9.12, 1.73, -10.0167) makes body 13 at (15.1333, 1.37, -39.15) in component "Display(ミラー)"
fillet "フィレット1'" radius 1.5 2 edges at (105, 42, 1) (105, 0, 1) on bodies 8 in component "SideUnit"
sketch "スケッチ14" plane through (0, 0, 210) normal (0, 0, 1) x (1, 0, 0) in component "SideUnit"
  line L0 (82, 40) -> (82, 24)
  line L1 (82, 24) -> (80, 24)
  line L2 (80, 24) -> (80, 22)
  line L3 (80, 22) -> (84, 22)
  line L4 (84, 22) -> (84, 42)
  line L5 (84, 42) -> (80, 42)
  line L6 (80, 42) -> (80, 40)
  line L7 (80, 40) -> (82, 40)
  line L8 (80, 22) -> (84, 22)
  line L9 (84, 22) -> (84, 15)
  line L10 (84, 15) -> (78, 15)
  circle A0 centre (81, 18.5) radius 1.6
  line L11 (81, 18.5) -> (81, 22) construction
  line L12 (80, 22) -> (78, 22)
  line L13 (78, 22) -> (78, 15)
  line L14 (81, 18.5) -> (81, 15) construction
  dimension "d171" = 3.2
  dimension "d172" = 3.5
  dimension "d173" = 7
  dimension "d231" = 6
  constraint coincident L3.end L4.start
  constraint perpendicular L8 L9
  constraint coincident A0.centre L11.start
  constraint perpendicular L3 L11
  constraint horizontal L10
  constraint coincident L2.end L3.start
  constraint perpendicular L2 L12
  constraint perpendicular L10 L13
  constraint coincident L10 L14.end
  constraint perpendicular L10 L14
  constraint midpoint L10 L14.end
  constraint coincident L8 L11.end
  measures "d171" diameter of A0
  measures "d172" distance of A0.centre L11.end
  measures "d173" distance of L3.end L9.end
  measures "d231" distance of L10.end L9.end
extrude "押し出し14" add sketch "スケッチ14" against normal blind 3 contours L3 L8 L9 L10 L12 L13 bodies 8 in component "SideUnit"
sketch "スケッチ15" plane through (80, 0, 0) normal (-1, 0, 0) x (0, 0, 1) in component "SideUnit"
  line L0 (2, 42) -> (2, 0)
  line L1 (2, 0) -> (52, 0)
  line L2 (52, 0) -> (52, 22)
  line L3 (52, 22) -> (138, 22)
  arc A0 (160, 0) -> (138, 22) centre (138, 0) ccw
  line L4 (160, 0) -> (170, 0)
  line L5 (170, 0) -> (170, 22)
  line L6 (170, 22) -> (207, 22)
  line L7 (207, 22) -> (210, 22)
  line L8 (210, 22) -> (210, 24)
  line L9 (210, 24) -> (168, 24)
  line L10 (168, 24) -> (168, 2)
  line L11 (168, 2) -> (161.9165, 2)
  arc A1 (161.9165, 2) -> (138, 24) centre (138, 0) ccw
  line L12 (138, 24) -> (50, 24)
  line L13 (50, 24) -> (50, 2)
  line L14 (50, 2) -> (30, 2)
  line L15 (30, 2) -> (30, 40)
  line L16 (30, 40) -> (210, 40)
  line L17 (210, 40) -> (210, 42)
  line L18 (210, 42) -> (2, 42)
  line L19 (30, 40) -> (20, 40)
  line L20 (20, 40) -> (20, 2)
  line L21 (20, 2) -> (30, 2)
  line L22 (30, 40) -> (30, 2)
  dimension "d232" = 10
  constraint coincident L15.end L16.start
  constraint perpendicular L15 L19
  constraint perpendicular L1 L20
  constraint coincident L14.end L15.start
  constraint horizontal L21
  measures "d232" distance of L20.end L14.end
extrude "押し出し15" cut sketch "スケッチ15" against normal up to surface (2 mm away) contours L15 L19 L20 L21 L22 bodies 8 in component "SideUnit"
mirror "コンポーネントをミラー化2" about plane through (0, 0, 0) normal (0, 0, 1) of bodies 8 makes body 14 in component "SideUnit(ミラー)"
ref_plane "作業平面1" through (0, 0, 210) normal (0, 0, 1) x (1, 0, 0) in component "BackUnit"
sketch "スケッチ1 (7)" plane through (0, 0, 210) normal (0, 0, 1) x (1, 0, 0) in component "BackUnit"
  line L0 (84, 42) -> (84, 15)
  line L1 (-84, 42) -> (-84, 15)
  line L2 (-84, 42) -> (84, 42)
  line L3 (-82, 40) -> (-82, 24)
  line L4 (-82, 40) -> (-80, 40)
  line L5 (82, 40) -> (80, 40)
  line L6 (82, 40) -> (82, 24)
  line L7 (-84, 15) -> (-84, 7)
  line L8 (-84, 7) -> (84, 7)
  line L9 (84, 7) -> (84, 15)
  line L10 (-82, 24) -> (-80, 24)
  line L11 (82, 24) -> (80, 24)
  line L12 (-80, 24) -> (-67, 24)
  line L13 (-67, 24) -> (-67, 40)
  line L14 (80, 24) -> (67, 24)
  line L15 (67, 24) -> (67, 40)
  circle A0 centre (81, 18.5) radius 1.6 construction
  line L16 (81, 20.1) -> (68.5, 20.1)
  arc A1 (68.5, 20.1) -> (68.5, 16.9) centre (68.5, 18.5) ccw
  line L17 (68.5, 16.9) -> (81, 16.9)
  arc A2 (81, 16.9) -> (81, 20.1) centre (81, 18.5) ccw
  line L18 (81, 18.5) -> (68.5, 18.5) construction
  line L19 (0, 42) -> (0, 7) construction
  line L20 (-68.5, 16.9) -> (-81, 16.9)
  arc A3 (-81, 20.1) -> (-81, 16.9) centre (-81, 18.5) ccw
  line L21 (-81, 20.1) -> (-68.5, 20.1)
  arc A4 (-68.5, 16.9) -> (-68.5, 20.1) centre (-68.5, 18.5) ccw
  line L22 (-80, 40) -> (-67, 40)
  line L23 (80, 40) -> (67, 40)
  circle A5 centre (-29, 36) radius 1.35
  circle A6 centre (29, 36) radius 1.35
  circle A7 centre (-29, 13) radius 1.35
  circle A8 centre (29, 13) radius 1.35
  line L24 (-29, 36) -> (29, 36) construction
  line L25 (29, 36) -> (29, 13) construction
  line L26 (29, 13) -> (-29, 13) construction
  line L27 (-29, 13) -> (-29, 36) construction
  line L28 (-29, 24.5) -> (29, 24.5) construction
  line L29 (-67, 40) -> (67, 40) construction
  line L30 (82, 24) -> (82, 8)
  line L31 (-82, 8) -> (-82, 24)
  line L32 (-29, 8) -> (-29, 7)
  line L33 (29, 8) -> (29, 7)
  line L34 (82, 8) -> (29, 8)
  line L35 (-29, 8) -> (-82, 8)
  circle A9 centre (-59, 24.5) radius 4.5
  line L36 (-29, 24.5) -> (-59, 24.5) construction
  line L37 (-57.3546, 27.35) -> (-60.6454, 27.35)
  line L38 (-60.6454, 27.35) -> (-62.2909, 24.5)
  line L39 (-62.2909, 24.5) -> (-60.6454, 21.65)
  line L40 (-60.6454, 21.65) -> (-57.3546, 21.65)
  line L41 (-57.3546, 21.65) -> (-55.7091, 24.5)
  line L42 (-55.7091, 24.5) -> (-57.3546, 27.35)
  circle A10 centre (59, 24.5) radius 4.5
  line L43 (60.6454, 27.35) -> (62.2909, 24.5)
  line L44 (57.3546, 27.35) -> (60.6454, 27.35)
  line L45 (55.7091, 24.5) -> (57.3546, 27.35)
  line L46 (57.3546, 21.65) -> (55.7091, 24.5)
  line L47 (60.6454, 21.65) -> (57.3546, 21.65)
  line L48 (62.2909, 24.5) -> (60.6454, 21.65)
  line L49 (-82, 21.35) -> (-67, 21.35)
  line L50 (-67, 21.35) -> (-67, 24)
  line L51 (-82, 15.65) -> (-67, 15.65)
  line L52 (-67, 15.65) -> (-67, 13.65)
  line L53 (-67, 13.65) -> (-82, 13.65)
  line L54 (82, 21.35) -> (67, 21.35)
  line L55 (67, 21.35) -> (67, 24)
  line L56 (82, 15.65) -> (67, 15.65)
  line L57 (67, 15.65) -> (67, 13.65)
  line L58 (67, 13.65) -> (82, 13.65)
  line L59 (82, 8) -> (83, 8)
  line L60 (83, 8) -> (83, 41)
  line L61 (83, 41) -> (-83, 41)
  line L62 (-83, 41) -> (-83, 8)
  line L63 (-83, 8) -> (-82, 8)
  line L64 (-82, 15.65) -> (-82, 13.65)
  line L65 (-82, 21.35) -> (-82, 24)
  line L66 (82, 21.35) -> (82, 24)
  line L67 (82, 15.65) -> (82, 13.65)
  circle A11 centre (-29, 36) radius 2.5
  circle A12 centre (-29, 13) radius 2.5
  circle A13 centre (29, 13) radius 2.5
  circle A14 centre (29, 36) radius 2.5
  point P0 (-59, 24.5)
  dimension "d176" = 15
  dimension "d177" = 15
  dimension "d178" = 3.2
  dimension "d179" = 12.5
  dimension "d180" = 35
  dimension "d183" = 2.7
  dimension "d184" = 58
  dimension "d185" = 23
  dimension "d189" = 1
  dimension "d190" = 9
  dimension "d191" = 30
  dimension "d193" = 5.7
  dimension "d200" = 2.85
  dimension "d201" = 2.85
  dimension "d202" = 2
  dimension "d216" = 1
  dimension "d217" = 1
  dimension "d218" = 1
  dimension "d219" = 5
  constraint coincident L1.start L2.start
  constraint coincident L0.start L2.end
  constraint coincident L1.end L7.start
  constraint parallel L1 L7
  constraint perpendicular L7 L8
  constraint coincident L0.end L9.end
  constraint vertical L9
  constraint coincident L10.end L12.start
  constraint perpendicular L3 L12
  constraint coincident L11.end L14.start
  constraint perpendicular L13 L14
  constraint tangent L16 A1
  constraint tangent A1 L17
  constraint parallel L16 L17
  constraint tangent L17 A2
  constraint tangent L16 A2
  constraint horizontal L18
  constraint coincident A0.centre A2.centre
  constraint midpoint L2 L19.start
  constraint midpoint L8 L19.end
  constraint symmetric L16.start L19 A3.start
  constraint symmetric L16.end L19 L21.end
  constraint symmetric A1.end L19 L20.start
  constraint symmetric L17.end L19 L20.end
  constraint symmetric A1 L19 A4
  constraint symmetric A2 L19 A3
  constraint coincident L4.end L22.start
  constraint perpendicular L13 L22
  constraint coincident L5.end L23.start
  constraint perpendicular L15 L23
  constraint equal A5 A6
  constraint equal A5 A7
  constraint equal A6 A8
  constraint coincident A5.centre L24.start
  constraint coincident A6.centre L24.end
  constraint perpendicular L19 L24
  constraint coincident A8.centre L25.end
  constraint perpendicular L24 L25
  constraint coincident A7.centre L26.end
  constraint perpendicular L25 L26
  constraint perpendicular L24 L27
  constraint midpoint L27 L28.start
  constraint midpoint L25 L28.end
  constraint midpoint L19 L28
  constraint coincident L6.end L11.start
  constraint perpendicular L29 L30
  constraint perpendicular L19 L34
  constraint coincident L3.end L10.start
  constraint vertical L31
  constraint coincident L32.start L34
  constraint coincident L8 L32.end
  constraint perpendicular L8 L32
  constraint coincident L8 L33.end
  constraint perpendicular L8 L33
  constraint collinear L34 L35
  constraint collinear L27 L32
  constraint collinear L25 L33
  constraint coincident P0 A9.centre
  constraint horizontal L36
  constraint horizontal L37
  constraint symmetric L19 A9 A10
  constraint symmetric L19 L37.start L44.start
  constraint symmetric L19 L37.end L43.start
  constraint symmetric L19 L38.end L43.end
  constraint symmetric L19 L39.end L47.start
  constraint symmetric L19 L40.end L46.start
  constraint symmetric L19 L41.end L45.start
  constraint coincident L31 L49.start
  constraint perpendicular L31 L49
  constraint vertical L50
  constraint coincident L31 L51.start
  constraint perpendicular L31 L51
  constraint equal L49 L51
  constraint perpendicular L51 L52
  constraint coincident L31 L53.end
  constraint perpendicular L31 L53
  constraint symmetric L12.end L19 L14.end
  constraint symmetric L19 L49.start L54.start
  constraint symmetric L19 L49.end L54.end
  constraint symmetric L19 L51.start L56.start
  constraint symmetric L19 L51.end L56.end
  constraint symmetric L19 L52.end L57.end
  constraint symmetric L19 L53.end L58.end
  constraint perpendicular L30 L59
  constraint perpendicular L34 L60
  constraint perpendicular L1 L61
  constraint perpendicular L2 L62
  constraint perpendicular L31 L63
  constraint concentric A5 A11
  constraint concentric A7 A12
  constraint concentric A8 A13
  constraint concentric A6 A14
  constraint equal A11 A12
  constraint equal A11 A14
  constraint equal A13 A14
  measures "d176" distance of L3 L13
  measures "d177" distance of L6 L15
  measures "d178" diameter of A1
  measures "d179" distance of A1.end L17.end
  measures "d180" distance of L2 L8
  measures "d183" diameter of A5
  measures "d184" distance of A5.centre A6.centre
  measures "d185" distance of A7.centre A5.centre
  measures "d189" distance of L8 L34
  measures "d190" diameter of A9
  measures "d191" distance of L27 P0
  measures "d193" distance of L39 L42
  measures "d200" distance of A3.centre L49
  measures "d201" distance of A3.centre L51
  measures "d202" distance of L51 L53
  measures "d216" distance of L2 L61
  measures "d217" distance of L1 L62
  measures "d218" distance of L0 L60
  measures "d219" diameter of A11
extrude "押し出し1'''''" add sketch "スケッチ1 (7)" along normal blind 1 separate body contours L0 L1 L2 L7 L8 L9 L32 L33 L34 L35 L59 L60 L61 L62 L63 | L8 L32 L33 L34 L35 L59 L60 L61 L62 L63 | L10 L12 L31 L49 L50 L65 | L11 L14 L30 L54 L55 L66 | A5 | A6 | A7 | A8 | L30 L56 L57 L58 L67 | L31 L51 L52 L53 L64 | A9 | L37 L38 L39 L40 L41 L42 | A10 | L43 L44 L45 L46 L47 L48 | A11 | A12 | A13 | A14 makes body 15 in component "BackUnit"
extrude "押し出し2'''" add sketch "スケッチ1 (7)" along normal blind 2 contours A11 | A12 | A13 | A14 bodies 15 in component "BackUnit"
extrude "押し出し3'''" add sketch "スケッチ1 (7)" along normal blind 3 contours L10 L12 L31 L49 L50 L65 | L11 L14 L30 L54 L55 L66 | L30 L56 L57 L58 L67 | L31 L51 L52 L53 L64 | A9 | A10 bodies 15 in component "BackUnit"
sketch "スケッチ2 (4)" plane through (0, 0, 212) normal (0, 0, 1) x (1, 0, 0) in component "BackUnitCover"
  line L0 (-84, 42) -> (84, 42)
  line L1 (-84, 42) -> (-84, 15)
  line L2 (-84, 15) -> (-84, 7)
  line L3 (-84, 7) -> (84, 7)
  line L4 (84, 42) -> (84, 15)
  line L5 (84, 7) -> (84, 15)
  circle A0 centre (-59, 24.5) radius 1.6
  circle A1 centre (59, 24.5) radius 1.6
  circle A2 centre (-29, 13) radius 1.35
  circle A3 centre (-29, 13) radius 2.5
  circle A4 centre (29, 13) radius 1.35
  circle A5 centre (29, 13) radius 2.5
  circle A6 centre (-29, 36) radius 1.35
  circle A7 centre (-29, 36) radius 2.5
  circle A8 centre (29, 36) radius 1.35
  circle A9 centre (29, 36) radius 2.5
  point P0 (59, 24.5)
  point P1 (-59, 24.5)
  dimension "d196" = 3.2
  constraint coincident P1 A0.centre
  constraint coincident P0 A1.centre
  constraint equal A0 A1
  measures "d196" diameter of A0
extrude "押し出し1''''''" add sketch "スケッチ2 (4)" along normal blind 1 separate body contours L0 L1 L2 L3 L4 L5 | A2 | A3 | A4 | A5 | A6 | A7 | A8 | A9 makes body 16 in component "BackUnitCover"
sketch "スケッチ1 (8)" plane through (0, 0, -3) normal (0, 0, -1) x (-1, 0, 0) in component "NosePart"
  line L0 (-7.1716, 40) -> (-7.1716, 2)
  line L1 (-7.1716, 2) -> (-7.1716, 0)
  line L2 (-7.1716, 0) -> (7.1716, 0)
  line L3 (7.1716, 0) -> (7.1716, 2)
  line L4 (7.1716, 2) -> (7.1716, 40)
  line L5 (7.1716, 42) -> (-7.1716, 42)
  line L6 (-7.1716, 42) -> (-7.1716, 40)
  line L7 (-7.1716, 0) -> (-7.1716, 2)
  line L8 (7.1716, 0) -> (7.1716, 2)
  line L9 (-7.1716, 2) -> (-7.1716, 10)
  line L10 (7.1716, 10) -> (7.1716, 2)
  line L11 (-7.1716, 10) -> (7.1716, 10)
  line L12 (-7.1716, 0) -> (-17.5, 0)
  line L13 (7.1716, 0) -> (17.5, 0)
  arc A0 (15, -15) -> (-15, -15) centre (0, -15) ccw
  line L14 (-15, -15) -> (-17.5, -15)
  line L15 (-17.5, -15) -> (-17.5, 0)
  line L16 (15, -15) -> (17.5, -15)
  line L17 (17.5, -15) -> (17.5, 0)
  line L18 (-15, -15) -> (-15, 0) construction
  line L19 (15, -15) -> (15, 0) construction
  line L20 (7.1716, 40) -> (7.1716, 42)
  dimension "d207" = 10
  dimension "d210" = 35
  dimension "d211" = 15
  constraint coincident L0.end L1.start
  constraint coincident L0 L9.end
  constraint parallel L0 L9
  constraint coincident L3 L10.start
  constraint coincident L3.end L4.start
  constraint parallel L8 L10
  constraint perpendicular L10 L11
  constraint coincident L1.end L2.start
  constraint perpendicular L7 L12
  constraint coincident L2.end L3.start
  constraint perpendicular L8 L13
  constraint coincident origin A0
  constraint horizontal L14
  constraint perpendicular L14 L15
  constraint horizontal L16
  constraint perpendicular L16 L17
  constraint equal L12 L13
  constraint equal L15 L17
  constraint equal L14 L16
  constraint coincident L12 L18.end
  constraint tangent A0 L18
  constraint perpendicular L12 L18
  constraint coincident L13 L19.end
  constraint tangent A0 L19
  measures "d207" distance of L11 L13
  measures "d210" distance of L15 L17
  measures "d211" distance of L16.end L13.end
extrude "押し出し1'''''''" add sketch "スケッチ1 (8)" along normal blind 3 separate body contours L0 L1 L2 L3 L4 L7 L8 L9 L10 L11 | L2 L12 A0 L14 L15 | L2 L13 A0 L16 L17 makes body 17 in component "NosePart"
extrude "押し出し2''''" add sketch "スケッチ1 (8)" against normal blind 3 contours L2 L12 A0 L14 L15 | L2 L13 A0 L16 L17 bodies 17 in component "NosePart"
sketch "スケッチ1 (9)" plane through (0, 0, 0) normal (0, 1, 0) x (1, 0, 0) in component "BoardPillar"
  circle A0 centre (0, 0) radius 1.25
  dimension "d220" = 2.5
  constraint coincident A0.centre origin
  measures "d220" diameter of A0
extrude "押し出し1''''''''" add sketch "スケッチ1 (9)" along normal blind 23 separate body makes body 18 in component "BoardPillar"
pattern_linear "206" [suppressed]
component "Display" placed x (0, 1, 0) y (-1, 0, 0) z (0, 0, 1) at (103, 7.825, -33.795)
component "Lens" placed x (0, 1, 0) y (-1, 0, 0) z (0, 0, 1) at (51.8703, 21, -24.5)
component "HalfMirror" placed x (0, -1, 0) y (0.707107, 0, 0.707107) z (-0.707107, 0, 0.707107) at (49.598, 40, -44.0122)
component "Pi Zero W" placed x (1, 0, 0) y (0, 0, 1) z (0, -1, 0) at (-32.5, 39.5, 213)